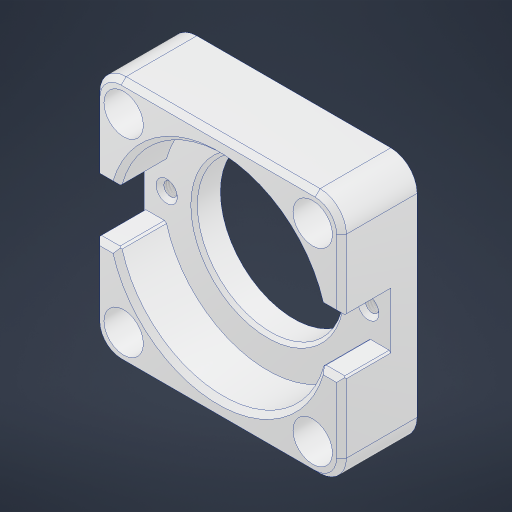
# Autodesk Inventor part: TH1-001
Saved by Autodesk Inventor 2024.3 (Build 283343000, 343)
## iProperties
Created: 2024-01-14
Part Number: TH1-001
Material: Aluminum 6061
Document SubType Name: Modeling
Designer: fablabadmin
Density: 2.7 g/cm^3
Appearance: Aluminum - Flat
Stock Number: SS4007
Description: Tool Holder base
Author: Benjamin Solar
Revision Number: 2
Autodesk Inventor part; units mm, degrees
ref_plane "YZ Plane" through (0, 0, 0) normal (1, 0, 0) x (0, 1, 0)
ref_plane "XZ Plane" through (0, 0, 0) normal (0, 1, 0) x (-1, 0, 0)
ref_plane "XY Plane" through (0, 0, 0) normal (0, 0, 1) x (1, 0, 0)
ref_plane "Work Plane1" through (31.775, 0, -7.95) normal (0, 0, -1) x (-1, 0, 0)
sketch "Sketch1" plane through (31.775, 0, -7.95) normal (0, 0, -1) x (-1, 0, 0)
  line L0 (62.5134, -8.05) -> (55.6, -8.05) construction
  line L1 (55.6, -8.05) -> (55.6, 8.05) construction
  line L2 (55.6, 8.05) -> (62.5134, 8.05) construction
  arc A0 (62.5134, 8.05) -> (1.0366, 8.05) centre (31.775, 0) ccw construction
  line L3 (1.0366, 8.05) -> (7.95, 8.05) construction
  line L4 (7.95, 8.05) -> (7.95, -8.05) construction
  line L5 (7.95, -8.05) -> (1.0366, -8.05) construction
  arc A1 (1.0366, -8.05) -> (62.5134, -8.05) centre (31.775, 0) ccw construction
  circle A2 centre (31.775, 0) radius 22.225 construction
  circle A3 centre (31.775, 0) radius 22.325
  line L6 (69.275, 37.5) -> (-5.725, 37.5)
  line L7 (-5.725, 37.5) -> (-5.725, -37.5)
  line L8 (-5.725, -37.5) -> (69.275, -37.5)
  line L9 (69.275, -37.5) -> (69.275, 37.5)
  line L10 (69.275, 37.5) -> (-5.725, -37.5) construction
  line L11 (-5.725, 37.5) -> (69.275, -37.5) construction
  dimension "d0" = 0.1
  dimension "d1" = 44.65
  dimension "d2" = 75
  constraints: 12 end point, 2 midpoint, 2 parallel, 2 perpendicular, 1 centre point, 1 coincident, 1 horizontal
  measures "d0" radial gap between concentric circles of A2 A3
  measures "d1" diameter of A3
  measures "d2" distance of L7.end L8.end
extrude "Extrusion1" add sketch "Sketch1" along normal blind 8
sketch "Sketch2" plane through (31.775, 0, -7.95) normal (0, 0, 1) x (1, 0, 0)
  line L0 (-62.5134, -8.05) -> (-55.6, -8.05) construction
  line L1 (-55.6, -8.05) -> (-55.6, 8.05) construction
  line L2 (-55.6, 8.05) -> (-62.5134, 8.05) construction
  arc A0 (-1.0366, 8.05) -> (-62.5134, 8.05) centre (-31.775, 0) ccw construction
  line L3 (-1.0366, 8.05) -> (-7.95, 8.05) construction
  line L4 (-7.95, 8.05) -> (-7.95, -8.05) construction
  line L5 (-7.95, -8.05) -> (-1.0366, -8.05) construction
  arc A1 (-62.5134, -8.05) -> (-1.0366, -8.05) centre (-31.775, 0) ccw construction
  circle A2 centre (-31.775, 0) radius 22.225 construction
  line L6 (5.725, 37.5) -> (5.725, -37.5) projected
  line L7 (-69.275, 37.5) -> (5.725, 37.5) projected
  line L8 (-69.275, -37.5) -> (-69.275, 37.5) projected
  line L9 (5.725, -37.5) -> (-69.275, -37.5) projected
  circle A3 centre (-31.775, 0) radius 22.325 construction
  circle A4 centre (-31.775, 0) radius 31.875
  line L10 (-55.6, -8.05) -> (-69.275, -8.05)
  line L11 (-69.275, -8.05) -> (-69.275, 8.05)
  line L12 (-69.275, 8.05) -> (-55.6, 8.05)
  line L13 (-55.6, 8.05) -> (-55.6, -8.05)
  line L14 (-84.275, 0) -> (20.725, 0) construction
  line L15 (-31.775, -52.5) -> (-31.775, 52.5) construction
  line L16 (-1.0366, -8.05) -> (-7.95, -8.05) construction
  line L17 (-7.95, -8.05) -> (-7.95, 8.05) construction
  line L18 (-7.95, 8.05) -> (-1.0366, 8.05) construction
  line L19 (-7.95, -8.05) -> (5.725, -8.05)
  line L20 (5.725, -8.05) -> (5.725, 8.05)
  line L21 (5.725, 8.05) -> (-7.95, 8.05)
  line L22 (-7.95, 8.05) -> (-7.95, -8.05)
  point P0 (-62.6167, 8.05)
  point P1 (-62.6167, -8.05)
  point P2 (-0.9333, 8.05)
  point P3 (5.725, 8.05)
  point P4 (5.725, -8.05)
  point P5 (-0.9333, -8.05)
  dimension "d7" = 0.1
  dimension "d9" = 0
  dimension "d29" = 0
  constraints: 22 end point, 4 symmetric about line, 2 parallel, 1 centre point, 1 coincident, 1 horizontal, 1 perpendicular, 1 point on line, 1 other
  measures "d7" radial gap between concentric circles of A1 A4
  measures "d9" distance between parallel lines of L1 L13
  measures "d29" distance between parallel lines of L0 L10
extrude "Extrusion2" add sketch "Sketch2" along normal blind 15 contours L6 L21 A4 L12 L8 L7 | L6 L9 L8 L10 A4 L19
sketch "Sketch3" plane through (31.775, 0, 7.05) normal (0, 0, 1) x (1, 0, 0)
  line L0 (-3.025, -28.75) -> (-60.525, -28.75)
  line L1 (-60.525, -28.75) -> (-60.525, 28.75)
  line L2 (-60.525, 28.75) -> (-3.025, 28.75)
  line L3 (-3.025, 28.75) -> (-3.025, -28.75)
  line L4 (-3.025, -28.75) -> (-60.525, 28.75) construction
  line L5 (-60.525, -28.75) -> (-3.025, 28.75) construction
  point P0 (-31.775, 0)
  dimension "d12" = 57.5
  constraints: 12 end point, 4 coincident, 2 midpoint, 2 parallel, 2 perpendicular, 1 horizontal
  measures "d12" distance of L1.end L2.end
hole "Hole1" at (-28.75, 28.75, 7.05) at (28.75, 28.75, 7.05) at (28.75, -28.75, 7.05) at (-28.75, -28.75, 7.05) direction (0, 0, -1) diameter 6.5 end through all counterbore diameter 12 counterbore depth 12
sketch "Sketch4" plane through (31.775, 0, -7.95) normal (0, 0, 1) x (1, 0, 0)
  circle A0 centre (-31.775, 0) radius 22.325 construction
  line L0 (5.725, 8.05) -> (-0.9333, 8.05) construction
  arc A1 (-0.9333, 8.05) -> (-62.6167, 8.05) centre (-31.775, 0) ccw construction
  line L1 (-62.6167, 8.05) -> (-69.275, 8.05) construction
  line L2 (-69.275, -8.05) -> (-69.275, 8.05) construction
  line L3 (-69.275, -8.05) -> (-62.6167, -8.05) construction
  arc A2 (-62.6167, -8.05) -> (-0.9333, -8.05) centre (-31.775, 0) ccw construction
  line L4 (-0.9333, -8.05) -> (5.725, -8.05) construction
  line L5 (5.725, 8.05) -> (5.725, -8.05) construction
  line L6 (5.725, 8.05) -> (-7.95, 8.05) construction
  line L7 (-7.95, -8.05) -> (5.725, -8.05) construction
  line L8 (5.725, -8.05) -> (5.725, 8.05) construction
  line L9 (-31.775, 0) -> (-9.45, 0) construction
  line L10 (-9.45, 0) -> (5.725, 0) construction
  line L11 (-1.1125, 8.05) -> (-1.1125, -8.05) construction
  line L12 (-0.9333, -8.05) -> (5.725, -8.05) construction
  line L13 (-31.775, -52.5) -> (-31.775, 52.5) construction
  line L14 (-7.95, -8.05) -> (-7.95, 8.05)
  line L15 (-7.95, 8.05) -> (-7.95, -8.05) projected
  point P0 (-1.1125, 0)
  point P1 (-62.4375, 0)
  dimension "d28" = 0
  constraints: 14 end point, 3 midpoint, 2 horizontal, 2 perpendicular, 1 horizontal alignment, 1 parallel, 1 point on line, 1 symmetric about line, 1 other
  measures "d28" distance between parallel lines of L15 L14
hole "Hole2" at (30.6625, 0, -7.95) at (-30.6625, 0, -7.95) direction (0, 0, -1) diameter 4.134 end through all countersink diameter 6.5 countersink angle 90 thread size "M5x0.8" class "6H" standard "ISO Metric profile"
fillet "Fillet1" radius 8 4 edges at (-37.5, -37.5, -4.45) (-37.5, 37.5, -4.45) (37.5, 37.5, -4.45) (37.5, -37.5, -4.45)
chamfer "Chamfer1" distance 1.5 angle 45 16 edges at (0, 31.875, 7.05) (0, -31.875, 7.05) (34.1709, 8.05, 7.05) (-34.1709, 8.05, 7.05) (-34.1709, -8.05, 7.05) (-37.5, -18.775, 7.05) (-35.1569, -35.1569, 7.05) (0, -37.5, 7.05) (35.1569, -35.1569, 7.05) (37.5, -18.775, 7.05) (-37.5, 18.775, 7.05) (-35.1569, 35.1569, 7.05) (0, 37.5, 7.05) (35.1569, 35.1569, 7.05) (37.5, 18.775, 7.05) (34.1709, -8.05, 7.05)
chamfer "Chamfer2" distance 1 angle 45 1 edges at (22.325, 0, -7.95)
chamfer "Chamfer3" distance 0.5 angle 45 6 edges at (-30.6625, 2.067, -15.95) (30.6625, 2.067, -15.95) (28.75, 32, -15.95) (-28.75, 32, -15.95) (-28.75, -25.5, -15.95) (28.75, -25.5, -15.95)
chamfer "Chamfer5" distance 0.5 angle 45 8 edges at (-30.8417, 8.05, -1.2) (30.8417, 8.05, -1.2) (-30.8417, -8.05, -1.2) (30.8417, -8.05, -1.2) (-37.5, 8.05, -1.2) (37.5, 8.05, -1.2) (37.5, -8.05, -1.2) (-37.5, -8.05, -1.2)
body "Solid1"
